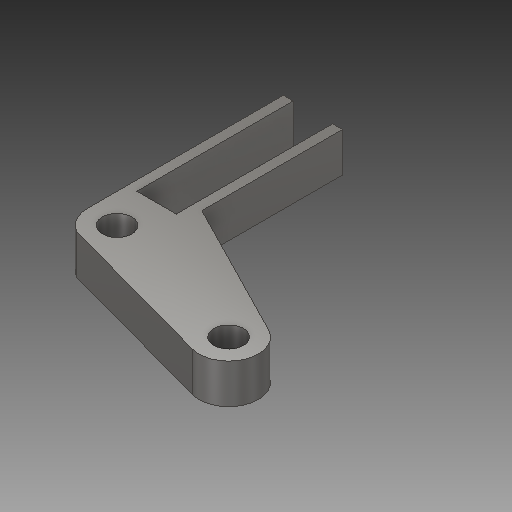
# Autodesk Inventor part: steeringarm
Saved by Autodesk Inventor 2018 (Build 220112000, 112)
## iProperties
Created: 2018-08-06
Part Number: steeringarm
Material: Steel, Mild
Document SubType Name: Modeling
Designer: Cole Tucker
Density: 7.85 g/cm^3
Appearance: Semi-Polished
Mass: 172.965 g
Surface Area: 89.1037 cm^2
Volume: 22.0337 cm^3
Author: Cole Tucker
Autodesk Inventor part; units mm, degrees
ref_plane "YZ Plane" through (0, 0, 0) normal (1, 0, 0) x (0, 1, 0)
ref_plane "XZ Plane" through (0, 0, 0) normal (0, 1, 0) x (-1, 0, 0)
ref_plane "XY Plane" through (0, 0, 0) normal (0, 0, 1) x (1, 0, 0)
sketch "Sketch1" plane through (0, 0, 0) normal (0, 1, 0) x (-1, 0, 0)
  line L0 (0, 0) -> (-50.8, 0) construction
  line L1 (0, 0) -> (-49.069, 13.148) construction
  arc A0 (-46.4918, 22.3177) -> (-53.8315, 4.8991) centre (-49.069, 13.148) ccw
  line L2 (0, 0) -> (0, -50.8) construction
  line L3 (9.525, 0) -> (9.525, -63.052)
  line L4 (-9.525, -63.052) -> (-9.525, -17.7513)
  arc A1 (9.525, 0) -> (4.7625, 8.2489) centre (0, 0) ccw
  line L5 (0, 0) -> (0, -12.7) construction
  circle A2 centre (0, 0) radius 4.7625
  circle A3 centre (-49.069, 13.148) radius 4.7625
  line L6 (6.35, -63.052) -> (9.525, -63.052)
  line L7 (-9.525, -63.052) -> (-6.35, -63.052)
  line L8 (0, -12.7) -> (6.35, -12.7)
  line L9 (6.35, -12.7) -> (6.35, -63.052)
  line L10 (0, -12.7) -> (-6.35, -12.7)
  line L11 (-6.35, -12.7) -> (-6.35, -63.052)
  line L12 (-53.8315, 4.8991) -> (-9.525, -17.7513)
  line L13 (4.7625, 8.2489) -> (-46.6038, 22.3485)
  dimension "d3" = 50.8
  dimension "d4" = 15
  dimension "d5" = 19.05
  dimension "d6" = 50.8
  dimension "d9" = 12.7
  dimension "d11" = 9.525
  dimension "d12" = 9.525
  dimension "d15" = 12.7
  dimension "d16" = 3.175
  dimension "d17" = 3.175
  constraints: 28 end point, 5 coincident, 5 point on circle, 4 centre point, 3 horizontal, 2 point on line, 2 vertical, 1 parallel, 1 perpendicular
  measures "d3" distance of L0.start L1.end
  measures "d4" angle of L0 L1
  measures "d5" diameter of A0
  measures "d6" distance of L0.start L2.end
  measures "d9" distance of L0.start L5.end
  measures "d11" diameter of A2
  measures "d12" diameter of A3
  measures "d15" distance between parallel lines of L9 L11
  measures "d16" distance of L6.start L3.end
  measures "d17" distance of L4.start L7.end
extrude "Extrusion1" add sketch "Sketch1" along normal blind 12.7
body "Solid1"
